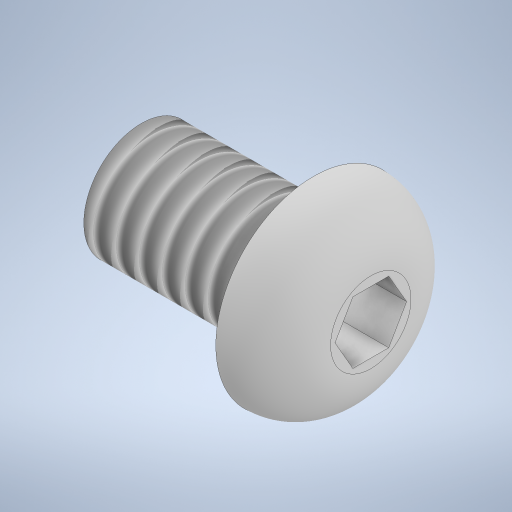
# Autodesk Inventor part: 1-4-20 screw
Saved by Autodesk Inventor 2024 (Build 280153000, 153)
## iProperties
Created: 2023-10-22
Part Number: 1-4-20 screw
Material: Generic
Document SubType Name: Modeling
Designer: olson
Density: 1 g/cm^3
Appearance: Default
Author: olson
Autodesk Inventor part; units mm, degrees
ref_plane "YZ Plane" through (0, 0, 0) normal (1, 0, 0) x (0, 1, 0)
ref_plane "XZ Plane" through (0, 0, 0) normal (0, 1, 0) x (-1, 0, 0)
ref_plane "XY Plane" through (0, 0, 0) normal (0, 0, 1) x (1, 0, 0)
sketch "Sketch1" plane through (0, 0, 0) normal (1, 0, 0) x (0, 1, 0)
  circle A0 centre (0, 0) radius 3.175
  dimension "d0" = 6.35
  constraints: 1 centre point, 1 coincident
  measures "d0" diameter of A0
extrude "Extrusion1" add sketch "Sketch1" along normal blind 9.525
sketch "Sketch2" plane through (9.525, 0, 0) normal (1, 0, 0) x (0, 0, -1)
  circle A0 centre (0, 0) radius 5.3975
  dimension "d3" = 10.795
  constraints: 1 centre point, 1 coincident
  measures "d3" diameter of A0
extrude "Extrusion2" add sketch "Sketch2" along normal blind 3.175
sketch "Sketch3" plane through (12.7, 0, 0) normal (1, 0, 0) x (0, 0, -1)
  line L0 (0, 0) -> (1.9812, 0)
  line L1 (0, 0) -> (-1.9812, 0)
  circle A0 centre (0, 0) radius 3.175 projected
  line L2 (0, 0) -> (0.9906, 1.7158)
  line L3 (0, 0) -> (1.9812, 0) construction
  line L4 (0.9906, 1.7158) -> (1.9812, 0)
  line L5 (0, 0) -> (-0.9906, 1.7158)
  line L6 (0, 0) -> (1.9812, 0) construction
  line L7 (-0.9906, 1.7158) -> (0.9906, 1.7158)
  line L8 (-0.9906, 1.7158) -> (-1.9812, 0)
  line L9 (0, 0) -> (0.9906, -1.7158)
  line L10 (0, 0) -> (1.9812, 0) construction
  line L11 (0.9906, -1.7158) -> (1.9812, 0)
  line L12 (0, 0) -> (-0.9906, -1.7158)
  line L13 (0, 0) -> (1.9812, 0) construction
  line L14 (-0.9906, -1.7158) -> (0.9906, -1.7158)
  line L15 (-0.9906, -1.7158) -> (-1.9812, 0)
  dimension "d6" = 1.9812
  dimension "d7" = 1.9812
  dimension "d8" = 1.9812
  dimension "d9" = 60
  dimension "d10" = 1.9812
  dimension "d11" = 120
  dimension "d12" = 1.9812
  dimension "d13" = 60
  dimension "d14" = 1.9812
  dimension "d15" = 120
  constraints: 32 end point, 6 horizontal, 4 equal length, 1 collinear
  measures "d6" distance of L0.start L0.end
  measures "d7" distance of L0.start L1.end
  measures "d8" distance of L2.start L2.end
  measures "d9" angle of L3 L2
  measures "d10" distance of L2.start L5.end
  measures "d11" angle of L6 L5
  measures "d12" distance of L2.start L9.end
  measures "d13" angle of L9 L10
  measures "d14" distance of L2.start L12.end
  measures "d15" angle of L12 L13
extrude "Extrusion3" cut sketch "Sketch3" against normal blind 3.175 contours L2 L4 L0 | L12 L15 L1 | L5 L7 L2 | L1 L8 L5 | L0 L11 L9 | L9 L14 L12
fillet "Fillet1" radius 3.175 1 edges at (12.7, 0, 5.3975)
thread "Thread1" size "1/4-20 UNC" class "2A" standard "ANSI Unified Screw Threads" full length
body "Solid1"
